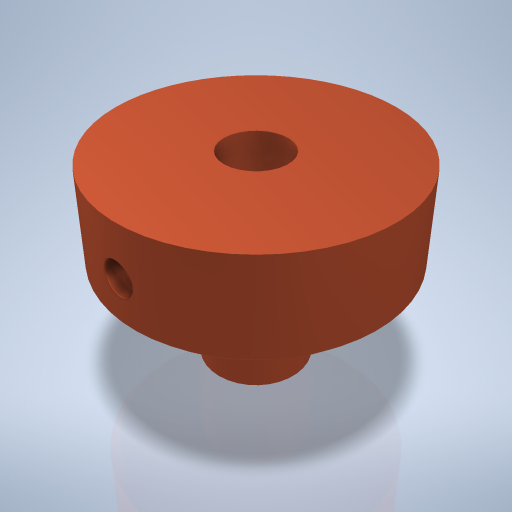
# Autodesk Inventor part: 30
Saved by Autodesk Inventor 2024.2 (Build 282272000, 272)
## iProperties
Created: 2024-05-14
Part Number: 30
Material: Kupfer
Document SubType Name: Modeling
Designer: Fabri
Density: 8.94 g/cm^3
Appearance: Kupfer - satiniert
Author: Fabri
Autodesk Inventor part; units mm, degrees
note: some values were not read from the file. Chosen so that the rebuilt part matches the saved one: direction of "Bohrung1".
ref_plane "YZ Plane" through (0, 0, 0) normal (1, 0, 0) x (0, 1, 0)
ref_plane "XZ Plane" through (0, 0, 0) normal (0, 1, 0) x (-1, 0, 0)
ref_plane "XY Plane" through (0, 0, 0) normal (0, 0, 1) x (1, 0, 0)
sketch "Skizze1" plane through (0, 0, 0) normal (0, 1, 0) x (-1, 0, 0)
  line L0 (0, 0) -> (14, 0)
  line L1 (14, 0) -> (14, -10)
  line L2 (14, -10) -> (5, -10)
  line L3 (5, -10) -> (5, -20)
  line L4 (5, -20) -> (0, -20)
  line L5 (0, -20) -> (0, 0)
  point P0 (9.5, -10)
  dimension "d0" = 10
  dimension "d1" = 10
  dimension "d2" = 10
  dimension "d3" = 28
  constraints: 12 end point, 5 perpendicular, 1 horizontal, 1 midpoint
  measures "d0" distance between parallel lines of L2 L0
  measures "d1" distance from line of L4 point (9.5, -10)
  measures "d2" diameter of L3 L5
  measures "d3" diameter of L1 L5
revolve "Umdrehung1" add sketch "Skizze1" angle 360 about axis through (0, 0, -20) along (0, 0, 1)
sketch "Skizze2" plane through (0, 0, 0) normal (0, 0, 1) x (1, 0, 0)
  circle A0 centre (0, 0) radius 14 projected
  point P0 (0, 0)
  constraints: 1 coincident
hole "Bohrung1" at (0, 0, 0) direction (0, 0, -1) diameter 6.5 depth 20
sketch "Skizze4" plane through (0, 0, 0) normal (0, 1, 0) x (-1, 0, 0)
  line L0 (-3.25, 0) -> (3.25, 0) projected
  point P0 (0, 0)
  point P1 (0, -5)
  dimension "d12" = 5
  constraints: 1 vertical alignment
  measures "d12" distance from line of point (0, -5) L0
hole "Bohrung2" at (0, 0, -5) direction (0, -1, 0) diameter 3.242 end through all thread size "M4x0.7" class "6H" standard "ISO Metric profile"
mirror "Spiegeln1" about plane through (0, 0, 0) normal (0, 1, 0) of "Bohrung2"
chamfer "Fasen1" distance 1 angle 45 1 edges at (14, 0, -10)
